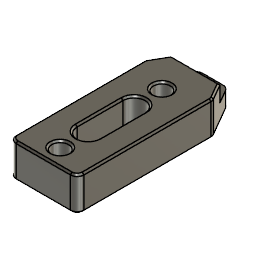
spannhalter_v2 (Autodesk Fusion 360 design; units mm, degrees)
part number: 2026-04-07-21-27-21-014
Autodesk Fusion 360 part; units mm, degrees
sketch "Skizze1" plane through (0, 0, 0) normal (0, 0, 1) x (1, 0, 0)
  line L0 (2, 0) -> (18, 0)
  line L1 (20, 2) -> (20, 39.4641)
  line L2 (13.0718, 50) -> (6.9282, 50)
  line L3 (0, 39.4641) -> (0, 2)
  line L4 (10, 50) -> (10, 0) construction
  circle A0 centre (10, 5) radius 2.5
  circle A1 centre (10, 35) radius 2.5
  line L5 (13.25, 26.75) -> (13.25, 13.25)
  line L6 (6.75, 13.25) -> (6.75, 26.75)
  arc A2 (13.25, 26.75) -> (6.75, 26.75) centre (10, 26.75) ccw
  arc A3 (6.75, 13.25) -> (13.25, 13.25) centre (10, 13.25) ccw
  line L7 (0, 40) -> (20, 40) construction
  line L8 (0.2679, 40.4641) -> (5.1962, 49)
  line L9 (19.7321, 40.4641) -> (14.8038, 49)
  line L10 (0, 45) -> (20, 45) construction
  line L11 (0, 26.75) -> (20, 26.75) construction
  line L12 (0, 13.25) -> (20, 13.25) construction
  line L13 (2.8868, 45) -> (17.1132, 45)
  arc A4 (0, 2) -> (2, 0) centre (2, 2) ccw
  arc A5 (18, 0) -> (20, 2) centre (18, 2) ccw
  arc A6 (0.2679, 40.4641) -> (0, 39.4641) centre (2, 39.4641) ccw
  arc A7 (20, 39.4641) -> (19.7321, 40.4641) centre (18, 39.4641) ccw
  arc A8 (14.8038, 49) -> (13.0718, 50) centre (13.0718, 48) ccw
  arc A9 (6.9282, 50) -> (5.1962, 49) centre (6.9282, 48) ccw
  point P0 (20, 0)
  point P1 (20, 40)
  dimension "breite" = 20
  dimension "loch_durchmesser" = 5
  dimension "d4" = 20
  dimension "d6" = 5
  dimension "d7" = 5
  dimension "d8" = 5
  dimension "d9" = 8.25
  dimension "d10" = 8.25
  dimension "kopf_lenge" = 10
  dimension "d13" = 10
  dimension "d14" = 60
  dimension "d15" = 60
  dimension "kopf_winkel" = 60
  dimension "d18" = 5
  dimension "d19" = 6.5
  dimension "d21" = 5
  dimension "d22" = 50
  dimension "d23" = 10
  dimension "d24" = 5
  dimension "parameter_1" = 2.5
  dimension "abrundung" = 2
  dimension "d27" = 2
  dimension "d28" = 2
  dimension "d29" = 2
  dimension "d30" = 2
  dimension "d31" = 2
  dimension "d32" = 2
  constraint horizontal L0
  constraint vertical L1
  constraint horizontal L2
  constraint vertical L3
  constraint parallel L1 L4
  constraint coincident L4 A0.centre
  constraint coincident L4 A1.centre
  constraint vertical L5
  constraint vertical L6
  constraint coincident L4 A2.centre
  constraint parallel L2 L7
  constraint coincident L1 P1
  constraint coincident L7 P1
  constraint parallel L2 L10
  constraint parallel L0 L11
  constraint parallel L0 L12
  constraint coincident L5.end L12
  constraint coincident L6.start L12
  constraint coincident L5.start L11
  constraint coincident L6.end L11
  constraint coincident A2.centre L11
  constraint coincident A3.centre L12
  constraint coincident L3 L11.start
  constraint coincident L3 L12.start
  constraint coincident L1 L12.end
  constraint coincident L1 L11.end
  constraint coincident L0 L4.end
  constraint coincident L2 L4.start
  constraint coincident origin L0
  constraint coincident origin L3
  constraint tangent L0 A4
  constraint tangent L3 A4
  constraint coincident P0 L0
  constraint coincident P0 L1
  constraint tangent L0 A5
  constraint tangent L1 A5
  constraint coincident L8 L13.start
  constraint coincident L3 L7.start
  constraint tangent L3 A6
  constraint tangent L8 A6
  constraint coincident L9 L13.end
  constraint coincident P1 L9
  constraint tangent L1 A7
  constraint tangent L9 A7
  constraint tangent L2 A8
  constraint tangent L9 A8
  constraint tangent L2 A9
  constraint tangent L8 A9
  constraint collinear L10 L13
  constraint equal L8 L9
  measures "d4" distance of origin P0
  measures "d6" diameter of A1
  measures "d7" diameter of A0
  measures "d8" distance of L0 A0.centre
  measures "d9" distance of A0.centre A3.centre
  measures "d10" distance of A1.centre A2.centre
  measures "d13" distance of L2 L7
  measures "d14" angle of L7 L9
  measures "d15" angle of L7 L8
  measures "d18" distance of L2 L10
  measures "d19" distance of L5 L6
  measures "d21" distance of P1 L10.end
  measures "d22" distance of L0 L2
  measures "d23" distance of L3 L4.end
  measures "d24" distance of A1.centre L7
  measures "d27" radius of A4
  measures "d28" radius of A5
  measures "d29" radius of A6
  measures "d30" radius of A9
  measures "d31" radius of A8
  measures "d32" radius of A7
extrude "Extrusion1" add sketch "Skizze1" against normal blind 10
extrude "Extrusion2" cut sketch "Skizze1" against normal blind 5 contours L2 L8 L9 L13 A8 A9
chamfer "Fase1" distance 0.5 angle 45 34 edges at (10, 30, 0) (13.25, 20, 0) (10, 10, 0) (6.75, 20, 0) (7.6692, 35.904, 0) (7.6692, 5.904, 0) (0, 20.7321, 0) (0.5858, 0.5858, 0) (10, 0, 0) (19.4142, 0.5858, 0) (20, 20.7321, 0) (19.9319, 39.9817, 0) (18.4226, 42.7321, 0) (1.5774, 42.7321, 0) (0.0681, 39.9817, 0) (10, 45, 0) (0, 20.7321, -10) (0.0681, 39.9817, -10) (2.7321, 44.7321, -10) (5.9282, 49.7321, -10) (10, 50, -10) (14.0718, 49.7321, -10) (17.2679, 44.7321, -10) (19.9319, 39.9817, -10) (20, 20.7321, -10) (19.4142, 0.5858, -10) (10, 0, -10) (0.5858, 0.5858, -10) (7.6692, 4.096, -10) (6.75, 20, -10) (10, 10, -10) (13.25, 20, -10) (10, 30, -10) (7.6692, 34.096, -10)
equation "breite = 20 mm"
equation "höhe = 50 mm"
equation "loch_durchmesser = 5 mm"
equation "d4 = breite"
equation "d6 = loch_durchmesser"
equation "d7 = loch_durchmesser"
equation "d8 = parameter_1 + loch_durchmesser / 2"
equation "d9 = ( öffnung_breite / 2 ) + ( loch_durchmesser / 2 ) + parameter_1"
equation "d10 = ( öffnung_breite / 2 ) + ( loch_durchmesser / 2 ) + parameter_1"
equation "kopf_lenge = 10 mm"
equation "d13 = kopf_lenge"
equation "d14 = kopf_winkel"
equation "d15 = kopf_winkel"
equation "kopf_winkel = 60 deg"
equation "d18 = kopf_lenge / 2"
equation "d19 = öffnung_breite"
equation "öffnung_breite = 6.50 mm"
equation "d21 = kopf_lenge / 2"
equation "d22 = höhe"
equation "d23 = breite / 2"
equation "d24 = parameter_1 + loch_durchmesser / 2"
equation "parameter_1 = 2.5 mm"
equation "abrundung = 2 mm"
equation "d27 = abrundung"
equation "d28 = abrundung"
equation "d29 = abrundung"
equation "d30 = abrundung"
equation "d31 = abrundung"
equation "d32 = abrundung"
